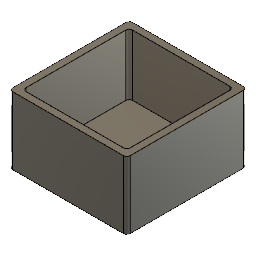
Case version 2 (Autodesk Fusion 360 design; units mm, degrees)
Autodesk Fusion 360 part; units mm, degrees
sketch "Sketch1" plane through (0, 0, 0) normal (0, 1, 0) x (1, 0, 0) in component "Case"
  line L0 (44.196, -45.085) -> (-44.196, -45.085)
  line L1 (-44.196, -45.085) -> (-44.196, 45.085)
  line L2 (-44.196, 45.085) -> (44.196, 45.085)
  line L3 (44.196, 45.085) -> (44.196, -45.085)
  line L4 (44.196, -45.085) -> (-44.196, 45.085) construction
  line L5 (-44.196, -45.085) -> (44.196, 45.085) construction
  dimension "d1" = 90.17
  dimension "d2" = 88.392
extrude "Extrude1" add sketch "Sketch1" along normal blind 50.8 makes body 1 in component "Case"
sketch "Sketch2" plane through (0, 50.8, 0) normal (0, 1, 0) x (-1, 0, 0) in component "Case"
  line L0 (-44.196, -45.085) -> (44.196, -45.085)
  line L1 (44.196, -45.085) -> (44.196, 45.085)
  line L2 (44.196, 45.085) -> (-44.196, 45.085)
  line L3 (-44.196, 45.085) -> (-44.196, -45.085)
sketch "Sketch3" plane through (0, 50.8, 0) normal (0, 1, 0) x (-1, 0, 0) in component "Case"
  line L0 (39.116, 40.005) -> (-39.116, 40.005)
  line L1 (-39.116, 40.005) -> (-39.116, -40.005)
  line L2 (-39.116, -40.005) -> (39.116, -40.005)
  line L3 (39.116, -40.005) -> (39.116, 40.005)
  line L4 (39.116, 40.005) -> (-39.116, -40.005) construction
  line L5 (-39.116, 40.005) -> (39.116, -40.005) construction
  dimension "d5" = 78.232
  dimension "d6" = 80.01
extrude "Extrude2" cut sketch "Sketch3" against normal blind 45.72 bodies 1 in component "Case"
fillet "Fillet1" radius 2.54 8 edges at (44.196, 25.4, 45.085) (-44.196, 25.4, 45.085) (39.116, 27.94, -40.005) (-39.116, 27.94, -40.005) (-44.196, 25.4, -45.085) (39.116, 27.94, 40.005) (-39.116, 27.94, 40.005) (44.196, 25.4, -45.085) on bodies 1 in component "Case"
sketch "Sketch5" plane through (0, 5.08, 0) normal (0, 1, 0) x (-1, 0, 0) in component "Case"
  circle A0 centre (-17.145, -22.225) radius 2.54
  circle A1 centre (-17.145, 22.225) radius 2.54
  circle A2 centre (21.336, 22.225) radius 2.54
  arc A3 (39.116, 37.465) -> (36.576, 40.005) centre (36.576, 37.465) ccw
  line L0 (36.576, 40.005) -> (-36.576, 40.005)
  arc A4 (-36.576, 40.005) -> (-39.116, 37.465) centre (-36.576, 37.465) ccw
  line L1 (-39.116, 37.465) -> (-39.116, -37.465)
  arc A5 (-39.116, -37.465) -> (-36.576, -40.005) centre (-36.576, -37.465) ccw
  line L2 (-36.576, -40.005) -> (36.576, -40.005)
  arc A6 (36.576, -40.005) -> (39.116, -37.465) centre (36.576, -37.465) ccw
  line L3 (39.116, -37.465) -> (39.116, 37.465)
  dimension "d19" = 5.08
  dimension "d20" = 5.08
  dimension "d21" = 5.08
  dimension "d22" = 17.145
  dimension "d23" = 17.145
  dimension "d24" = 21.336
  dimension "d25" = 22.225
  dimension "d26" = 22.225
  dimension "d27" = 22.225
  measures "d19" diameter of A0
  measures "d20" diameter of A1
  measures "d21" diameter of A2
  measures "d22" distance of origin
  measures "d23" distance of origin
  measures "d26" distance of origin
  measures "d27" distance of origin
sketch "Sketch6" plane through (0, 5.08, 0) normal (0, 1, 0) x (-1, 0, 0) in component "Case"
  circle A0 centre (-17.145, 22.225) radius 2.54
  arc A1 (39.116, 37.465) -> (36.576, 40.005) centre (36.576, 37.465) ccw
  line L0 (36.576, 40.005) -> (-36.576, 40.005)
  arc A2 (-36.576, 40.005) -> (-39.116, 37.465) centre (-36.576, 37.465) ccw
  line L1 (-39.116, 37.465) -> (-39.116, -37.465)
  arc A3 (-39.116, -37.465) -> (-36.576, -40.005) centre (-36.576, -37.465) ccw
  line L2 (-36.576, -40.005) -> (36.576, -40.005)
  arc A4 (36.576, -40.005) -> (39.116, -37.465) centre (36.576, -37.465) ccw
  line L3 (39.116, -37.465) -> (39.116, 37.465)
  dimension "d30" = 5.08
  dimension "d31" = 17.145
  dimension "d32" = 22.225
  measures "d30" diameter of A0
  measures "d31" distance of origin
extrude "Extrude4" add sketch "Sketch6" along normal blind 15.24 separate body contours A0 makes body 2 in component "Case"
sketch "Sketch7" plane through (0, 5.08, 0) normal (0, 1, 0) x (-1, 0, 0) in component "Case"
  arc A0 (39.116, 37.465) -> (36.576, 40.005) centre (36.576, 37.465) ccw
  line L0 (36.576, 40.005) -> (-36.576, 40.005)
  arc A1 (-36.576, 40.005) -> (-39.116, 37.465) centre (-36.576, 37.465) ccw
  line L1 (-39.116, 37.465) -> (-39.116, -37.465)
  arc A2 (-39.116, -37.465) -> (-36.576, -40.005) centre (-36.576, -37.465) ccw
  line L2 (-36.576, -40.005) -> (36.576, -40.005)
  arc A3 (36.576, -40.005) -> (39.116, -37.465) centre (36.576, -37.465) ccw
  line L3 (39.116, -37.465) -> (39.116, 37.465)
  circle A4 centre (21.336, 22.225) radius 2.54
  dimension "d35" = 5.08
  dimension "d36" = 21.336
  dimension "d37" = 22.225
  measures "d35" diameter of A4
extrude "Extrude5" add sketch "Sketch7" along normal blind 15.24 contours A4 bodies 1 in component "Case"
sketch "Sketch8" plane through (0, 5.08, 0) normal (0, 1, 0) x (-1, 0, 0) in component "Case"
  circle A0 centre (21.336, 22.225) radius 2.54
  arc A1 (39.116, 37.465) -> (36.576, 40.005) centre (36.576, 37.465) ccw
  line L0 (36.576, 40.005) -> (-36.576, 40.005)
  arc A2 (-36.576, 40.005) -> (-39.116, 37.465) centre (-36.576, 37.465) ccw
  line L1 (-39.116, 37.465) -> (-39.116, -37.465)
  arc A3 (-39.116, -37.465) -> (-36.576, -40.005) centre (-36.576, -37.465) ccw
  line L2 (-36.576, -40.005) -> (36.576, -40.005)
  arc A4 (36.576, -40.005) -> (39.116, -37.465) centre (36.576, -37.465) ccw
  line L3 (39.116, -37.465) -> (39.116, 37.465)
  circle A5 centre (-17.145, -22.225) radius 2.54
  dimension "d40" = 5.08
  dimension "d41" = 22.225
  dimension "d42" = 17.145
  measures "d40" diameter of A5
  measures "d41" distance of origin
  measures "d42" distance of origin
extrude "Extrude6" add sketch "Sketch8" along normal blind 15.24 contours A5 bodies 1 in component "Case"
sketch "Sketch9" plane through (0, 20.32, 0) normal (0, 1, 0) x (-1, 0, 0) in component "Case"
  circle A0 centre (-17.145, 22.225) radius 2.54
  circle A1 centre (-17.145, 22.225) radius 1.1938
  dimension "d45" = 2.3876
  measures "d45" diameter of A1
extrude "Extrude7" cut sketch "Sketch9" against normal blind 7.62 contours A1 bodies 2 in component "Case"
sketch "Sketch10" plane through (0, 20.32, 0) normal (0, 1, 0) x (-1, 0, 0) in component "Case"
  circle A0 centre (21.336, 22.225) radius 2.54
  circle A1 centre (21.336, 22.225) radius 1.1938
  dimension "d48" = 2.3876
  measures "d48" diameter of A1
extrude "Extrude8" cut sketch "Sketch10" against normal blind 7.62 contours A1 bodies 1 in component "Case"
sketch "Sketch11" plane through (0, 20.32, 0) normal (0, 1, 0) x (-1, 0, 0) in component "Case"
  circle A0 centre (-17.145, -22.225) radius 2.54
  circle A1 centre (-17.145, -22.225) radius 1.1938
  dimension "d51" = 2.3876
  measures "d51" diameter of A1
extrude "Extrude9" cut sketch "Sketch11" against normal blind 7.62 contours A1 bodies 1 in component "Case"
component "Case" placed x (1, 0, 0) y (0, 1, 0) z (0, 0, 1) at (0, 0, 0)
